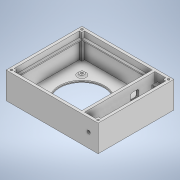
# Autodesk Inventor part: mainBody
Saved by Autodesk Inventor 2021 (Build 250183000, 183)
## iProperties
Created: 2021-04-02
Part Number: mainBody
Material: Generic
Document SubType Name: Modeling
Designer: awitc
Density: 1 g/cm^3
Appearance: Default
Author: awitc
Autodesk Inventor part; units mm, degrees
ref_plane "YZ Plane" through (0, 0, 0) normal (1, 0, 0) x (0, 1, 0)
ref_plane "XZ Plane" through (0, 0, 0) normal (0, 1, 0) x (-1, 0, 0)
ref_plane "XY Plane" through (0, 0, 0) normal (0, 0, 1) x (1, 0, 0)
sketch "Sketch1" plane through (0, 0, 0) normal (0, 1, 0) x (-1, 0, 0)
  circle A0 centre (76, 0) radius 2.25
  circle A1 centre (76, -76) radius 2.25
  circle A2 centre (0, 0) radius 2.25
  circle A3 centre (0, -76) radius 2.25
  circle A4 centre (38, -38) radius 41
  line L0 (103, 18) -> (103, 27)
  line L1 (103, 27) -> (94, 27)
  line L2 (103, 27) -> (-27, 27)
  line L3 (-27, 27) -> (-27, -103)
  line L4 (-27, -103) -> (103, -103)
  line L5 (103, -103) -> (103, 27)
  line L6 (108, 27) -> (108, 32)
  line L7 (108, 32) -> (103, 32)
  line L8 (108, 32) -> (-32, 32)
  line L9 (-32, 32) -> (-32, -108)
  line L10 (-32, -108) -> (108, -108)
  line L11 (108, -108) -> (108, 32)
  line L12 (-32, 32) -> (-62, 32)
  line L13 (-62, 32) -> (-62, -108)
  line L14 (-62, -108) -> (-32, -108)
  line L15 (-32, -108) -> (-32, 32)
  line L16 (-32, 27) -> (-57, 27)
  line L17 (-57, 27) -> (-57, -103)
  line L18 (-57, -103) -> (-32, -103)
  dimension "d3" = 4.5
  dimension "d4" = 4.5
  dimension "d5" = 4.5
  dimension "d10" = 82
  dimension "d41" = 130
  dimension "d42" = 130
  dimension "d51" = 5
  dimension "d52" = 5
  dimension "d53" = 140
  dimension "d54" = 140
  dimension "d57" = 30
  dimension "d58" = 25
  constraints: 38 end point, 6 parallel, 6 perpendicular, 5 centre point, 3 horizontal, 2 point on line, 1 coincident
  measures "d3" diameter of A1
  measures "d4" diameter of A2
  measures "d5" diameter of A3
  measures "d10" diameter of A4
  measures "d41" distance of L4.end L3.end
  measures "d42" distance of L3.end L2.end
  measures "d51" distance of L7.end L6.end
  measures "d52" distance of L6.end L6.start
  measures "d53" distance of L10.end L9.end
  measures "d54" distance of L9.end L8.end
  measures "d57" distance of L14.end L13.end
  measures "d58" distance of L16.start L16.end
extrude "Extrusion3" add sketch "Sketch1" along normal blind 3 contours L5 L4 L3 L2 L1 L0 | L18 L17 L16 L9
extrude "Extrusion5" add sketch "Sketch1" along normal blind 36.5 contours L11 L10 L9 L8 L7 L6 | L14 L13 L12 L9 L16 L17 L18
sketch "Sketch4" plane through (0, 3, 0) normal (0, 1, 0) x (1, 0, 0)
  circle A0 centre (-38, 38) radius 41 projected
  circle A1 centre (-38, 38) radius 41
  circle A2 centre (-38, 38) radius 42
  circle A3 centre (-76, 0) radius 2.25 projected
  circle A4 centre (-76, 0) radius 5
  circle A5 centre (-76, 76) radius 2.25 projected
  circle A6 centre (-76, 76) radius 5
  circle A7 centre (0, 76) radius 5
  circle A8 centre (0, 0) radius 5
  circle A9 centre (0, 0) radius 2.25 projected
  circle A10 centre (0, 0) radius 2.25
  circle A11 centre (0, 76) radius 2.25
  dimension "d59" = 84
  dimension "d78" = 10
  dimension "d79" = 10
  dimension "d80" = 10
  dimension "d81" = 10
  constraints: 8 centre point, 7 coincident
  measures "d59" diameter of A2
  measures "d78" diameter of A4
  measures "d79" diameter of A6
  measures "d80" diameter of A7
  measures "d81" diameter of A8
extrude "Extrusion6" cut sketch "Sketch4" against normal blind 1 contours A2
sketch "Sketch5" plane through (32, 3, -103) normal (1, 0, 0) x (0, 0, -1)
  line L0 (-130, 0) -> (0, 0) projected
  line L1 (-130, 33.5) -> (0, 33.5) projected
  line L2 (0, 0) -> (-30, 0)
  line L3 (-30, 0) -> (-30, 33.5)
  line L4 (-30, 33.5) -> (0, 33.5)
  line L5 (0, 33.5) -> (0, 0)
  line L6 (-30, 33.5) -> (-45, 33.5)
  line L7 (-45, 33.5) -> (-45, 18.5)
  line L8 (-45, 18.5) -> (-30, 18.5)
  line L9 (-30, 18.5) -> (-30, 33.5)
  point P0 (-103, -3)
  point P1 (-30, 18.5)
  dimension "d62" = 30
  dimension "d63" = 15
  dimension "d64" = 15
  constraints: 16 end point, 4 parallel, 2 horizontal, 2 perpendicular, 1 point on line
  measures "d62" distance of L3.end L4.end
  measures "d63" distance of L8.end L7.end
  measures "d64" distance of L7.end L6.end
extrude "Extrusion7" cut sketch "Sketch5" against normal up to surface (5 mm away) contours L8 L7 L1 L3
fillet "Fillet1" radius 2 2 edges at (29.5, 21.5, -58) (29.5, 21.5, -73)
sketch "Sketch6" plane through (0, 36.5, 0) normal (0, 1, 0) x (1, 0, 0)
  line L0 (-108, 108) -> (-108, -32) projected
  line L1 (62, 108) -> (-108, 108) projected
  line L2 (-108, -32) -> (32, -32)
  line L3 (32, -27) -> (32, 103)
  line L4 (32, 108) -> (-108, 108)
  line L5 (-108, 108) -> (-108, -32)
  line L6 (-103, -27) -> (-103, 103) projected
  line L7 (-103, 103) -> (27, 103) projected
  line L8 (-103, -27) -> (27, -27)
  line L9 (27, -27) -> (27, 103)
  line L10 (27, 103) -> (-103, 103)
  line L11 (-103, 103) -> (-103, -27)
  line L12 (-103, -27) -> (27, -27) projected
  line L13 (-103, -27) -> (-98, -27)
  line L14 (-103, -22) -> (-103, -27)
  line L15 (-98, -22) -> (22, -22)
  line L16 (22, -22) -> (22, 98)
  line L17 (22, 98) -> (-98, 98)
  line L18 (-98, 98) -> (-98, -22)
  line L19 (32, -32) -> (62, -32)
  line L20 (62, -32) -> (62, -27)
  line L21 (57, -27) -> (32, -27)
  line L22 (62, 108) -> (-108, 108) projected
  line L23 (57, -27) -> (57, 103)
  line L24 (57, 108) -> (62, 108)
  line L25 (62, 108) -> (62, -27)
  line L26 (32, 103) -> (57, 103)
  line L27 (57, 108) -> (32, 108)
  point P0 (0, 0)
  dimension "d68" = 140
  dimension "d69" = 5
  dimension "d71" = 120
  dimension "d72" = 120
  dimension "d75" = 5
  constraints: 44 end point, 9 parallel, 6 horizontal, 4 perpendicular, 2 point on line
  measures "d68" distance of L4.end L4.start
  measures "d69" distance of L14.start L15.start
  measures "d71" distance of L17.end L16.end
  measures "d72" distance of L16.end L15.end
  measures "d75" distance of L24.start L24.end
extrude "Extrusion8" add sketch "Sketch6" along normal blind 2 contours L6 L7 L9 L8
extrude "Extrusion9" add sketch "Sketch6" along normal blind 12.5 contours L1 L25 L20 L19 L2 L0
extrude "Extrusion10" add sketch "Sketch4" along normal blind 3 contours A4 | A6 | A7 | A8
sketch "Sketch7" plane through (0, 0, 0) normal (0, -1, 0) x (1, 0, 0)
  circle A0 centre (-76, 0) radius 4.5
  circle A1 centre (0, 0) radius 4.5
  circle A2 centre (0, -76) radius 4.5
  circle A3 centre (-76, -76) radius 4.5
  dimension "d153" = 9
  dimension "d154" = 9
  dimension "d156" = 9
  constraints: 4 centre point, 4 coincident
  measures "d153" diameter of A0
  measures "d154" diameter of A1
  measures "d156" diameter of A3
extrude "Extrusion11" cut sketch "Sketch7" against normal blind 3
sketch "Sketch8" plane through (57, 3, 27) normal (0, 0, -1) x (-1, 0, 0)
  line L0 (25, 0) -> (0, 0) projected
  line L1 (12.5, 0) -> (12.5, 23)
  circle A0 centre (12.5, 23) radius 3
  point P0 (57, -3)
  dimension "d91" = 23
  dimension "d92" = 6
  constraints: 2 end point, 1 centre point, 1 coincident, 1 midpoint, 1 vertical
  measures "d91" distance of L1.start L1.end
  measures "d92" diameter of A0
extrude "Extrusion12" cut sketch "Sketch8" against normal up to surface (5 mm away)
sketch "Sketch9" plane through (32, 3, -103) normal (0, 0, 1) x (1, 0, 0)
  circle A0 centre (12.5, 23) radius 3 projected
  circle A1 centre (12.5, 23) radius 5
  line L0 (6.5, 23) -> (6.5, 30)
  line L1 (6.5, 30) -> (12.5, 30)
  line L2 (6.5, 30) -> (18.5, 30)
  line L3 (18.5, 30) -> (18.5, 16)
  line L4 (18.5, 16) -> (6.5, 16)
  line L5 (6.5, 16) -> (6.5, 30)
  line L6 (4.5, 16) -> (4.5, 14)
  line L7 (4.5, 14) -> (6.5, 14)
  line L8 (4.5, 14) -> (20.5, 14)
  line L9 (20.5, 14) -> (20.5, 32)
  line L10 (20.5, 32) -> (4.5, 32)
  line L11 (4.5, 32) -> (4.5, 14)
  point P0 (-32, -3)
  point P1 (4.5, 16)
  dimension "d95" = 10
  dimension "d99" = 6
  dimension "d100" = 7
  dimension "d102" = 14
  dimension "d103" = 2
  dimension "d104" = 2
  dimension "d105" = 16
  dimension "d106" = 18
  constraints: 24 end point, 4 parallel, 2 horizontal, 2 perpendicular, 1 centre point, 1 coincident
  measures "d95" diameter of A1
  measures "d99" distance of L0.end L1.end
  measures "d100" distance of L0.start L0.end
  measures "d102" distance of L2.end L3.end
  measures "d103" distance of L7.end L6.end
  measures "d104" distance of L6.end L6.start
  measures "d105" distance of L10.end L9.end
  measures "d106" distance of L9.end L8.end
extrude "Extrusion13" cut sketch "Sketch9" against normal up to surface (5 mm away) contours A0 | A1
extrude "Extrusion14" add sketch "Sketch9" along normal blind 10 contours L11 L10 L9 L8 L7 L6
draft "FaceDraft1" angle 5 pull direction (0, 0, 1) faces at (38.5, 23.6667, -99.6667) (46.5, 19, -96.3333) (50.5, 28.3333, -99.6667) (42.5, 33, -96.3333) fixed edges at (38.5, 26, -93) (44.5, 19, -93) (50.5, 26, -93) (44.5, 33, -93)
sketch "Sketch12" plane through (32, 3, -103) normal (0, 0, 1) x (1, 0, 0)
  line L0 (4.5, 32) -> (4.5, 14) projected
  line L1 (4.5, 14) -> (20.5, 14)
  line L2 (20.5, 14) -> (20.5, 0)
  line L3 (20.5, 0) -> (4.5, 0)
  line L4 (4.5, 0) -> (4.5, 14)
  line L5 (4.5, 0) -> (6.5, 0)
  line L6 (25, 0) -> (0, 0) projected
  line L7 (6.5, 0) -> (6.5, 14)
  line L8 (20.5, 0) -> (18.5, 0)
  line L9 (18.5, 0) -> (18.5, 14)
  line L10 (12.5, 0) -> (13.5, 0)
  line L11 (12.5, 0) -> (11.5, 0)
  line L12 (11.5, 0) -> (13.5, 0)
  line L13 (13.5, 0) -> (13.5, 14)
  line L14 (13.5, 14) -> (11.5, 14)
  line L15 (11.5, 14) -> (11.5, 0)
  point P0 (-32, -3)
  point P1 (11.5, 14)
  point P2 (11.5, 0)
  point P3 (13.5, 0)
  point P4 (13.5, 14)
  point P5 (6.5, 0)
  dimension "d135" = 16
  dimension "d136" = 14
  dimension "d137" = 2
  dimension "d138" = 2
  dimension "d139" = 14
  dimension "d140" = 1
  dimension "d141" = 1
  dimension "d142" = 14
  constraints: 28 end point, 6 point on line, 4 parallel, 3 perpendicular, 2 horizontal, 1 midpoint
  measures "d135" distance of L2.end L3.end
  measures "d136" distance of L1.end L2.end
  measures "d137" distance of L3.end L5.end
  measures "d138" distance of L2.end L8.end
  measures "d139" distance of L8.end L9.end
  measures "d140" distance of L10.start L10.end
  measures "d141" distance of L10.start L11.end
  measures "d142" distance of L13.end L12.end
extrude "Extrusion17" add sketch "Sketch12" along normal blind 10 contours L1 L7 L3 L4 | L1 L13 L3 L15 | L1 L2 L3 L9
sketch "Sketch14" plane through (-38, 2, -38) normal (0, 1, 0) x (1, 0, 0)
  circle A0 centre (0, 0) radius 41
  circle A1 centre (0, 0) radius 42
  point P0 (38, -38)
  constraints: 2 centre point, 1 coincident
extrude "Extrusion19" cut sketch "Sketch14" against normal blind 1
fillet "Fillet4" radius 5 5 edges at (27, 36.5, -88) (-38, 36.5, -103) (-103, 36.5, -38) (-38, 36.5, 27) (27, 36.5, -15.5)
fillet "Fillet5" radius 3 2 edges at (24.5, 36.5, -73) (24.5, 36.5, -58)
fillet "Fillet6" radius 3 4 edges at (-81, 3, -76) (-5, 3, -76) (-5, 3, 0) (-81, 3, 0)
sketch "Sketch15" plane through (0, 49, 0) normal (0, 1, 0) x (1, 0, 0)
  line L0 (-103, -27) -> (-103, 103) projected
  line L1 (-98, -22) -> (-98, 98) projected
  line L2 (-103, 103) -> (-98, 103)
  line L3 (-98, 103) -> (-98, 98)
  line L4 (-98, 98) -> (-103, 98)
  line L5 (-103, 98) -> (-103, 103)
  line L6 (27, 103) -> (27, 73) projected
  line L7 (27, 103) -> (22, 103)
  line L8 (22, 103) -> (22, 98)
  line L9 (22, 98) -> (27, 98)
  line L10 (27, 98) -> (27, 103)
  line L11 (27, -27) -> (27, 103) projected
  line L12 (22, -22) -> (-98, -22) projected
  line L13 (27, -27) -> (22, -27)
  line L14 (22, -27) -> (22, -22)
  line L15 (22, -22) -> (27, -22)
  line L16 (27, -22) -> (27, -27)
  line L17 (-103, -27) -> (-98, -27)
  line L18 (-98, -27) -> (-98, -22)
  line L19 (-98, -22) -> (-103, -22)
  line L20 (-103, -22) -> (-103, -27)
  line L21 (-103, -27) -> (-103, 103) projected
  circle A0 centre (-103, 103) radius 2
  line L22 (27, 103) -> (27, -27) projected
  circle A1 centre (27, 103) radius 2
  line L23 (27, -27) -> (-103, -27) projected
  circle A2 centre (27, -27) radius 2
  circle A3 centre (-103, -27) radius 2
  line L24 (57, -27) -> (57, 103) projected
  line L25 (57, 103) -> (52, 103)
  line L26 (52, 103) -> (52, 98)
  line L27 (52, 98) -> (57, 98)
  line L28 (57, 98) -> (57, 103)
  line L29 (57, -27) -> (32, -27) projected
  line L30 (57, -27) -> (52, -27)
  line L31 (52, -27) -> (52, -22)
  line L32 (52, -22) -> (57, -22)
  line L33 (57, -22) -> (57, -27)
  circle A4 centre (57, -27) radius 2
  circle A5 centre (57, 103) radius 2
  point P0 (0, 0)
  point P1 (27, 101)
  point P2 (25, 103)
  point P3 (-103, -25)
  point P4 (-101, -27)
  point P5 (25, -27)
  point P6 (27, -25)
  point P7 (-101, 103)
  point P8 (-103, 101)
  point P9 (55, -27)
  point P10 (57, -25)
  point P11 (57, 101)
  point P12 (55, 103)
  dimension "d157" = 4
  dimension "d158" = 4
  dimension "d159" = 4
  dimension "d160" = 4
  dimension "d165" = 5
  dimension "d166" = 4
  dimension "d167" = 4
  constraints: 48 end point, 12 parallel, 6 centre point, 6 coincident, 6 horizontal, 6 perpendicular, 2 point on line
  measures "d157" diameter of A0
  measures "d158" diameter of A1
  measures "d159" diameter of A2
  measures "d160" diameter of A3
  measures "d165" distance of L27.end L26.end
  measures "d166" diameter of A4
  measures "d167" diameter of A5
extrude "Extrusion21" add sketch "Sketch15" against normal blind 47 contours L19 L18 L17 A3 L0 | L0 A0 L2 L3 L4 | A3 L17 L0 | L0 L2 A0 | L29 A4 L24 | A4 L29 L31 L32 L24 | L27 L26 L25 A5 L24 | A5 L25 L24 picked at (-102.2951, -25.8781) picked at (-102.5624, 101.7494) picked at (55.6834, -26.8517) picked at (56.8517, 101.6834)
extrude "Extrusion22" cut sketch "Sketch15" against normal blind 20 contours A3 L17 L0 | L0 L17 A3 | A0 L2 L0 | L0 L2 A0 | L29 A4 L24 | L24 A4 L29 | A5 L25 L24 | L24 L25 A5
body "Solid3"
